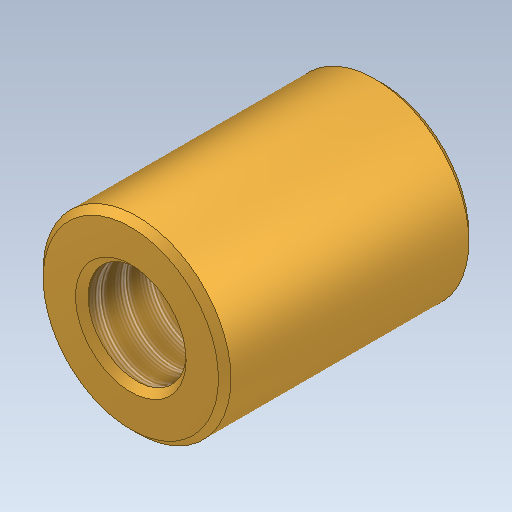
# Autodesk Inventor part: SB-203040
Saved by Autodesk Inventor 2021 (Build 250183000, 183)
## iProperties
Created: 2020-09-13
Part Number: SB-203040
Material: 真鍮、ソフト イエロー
Document SubType Name: Modeling
Designer: Yuta Kage
Mass: 0.173147 g
Surface Area: 0.662651 cm^2
Volume: 0.0204424 cm^3
Density: 8.47 g/cm^3
Appearance: 真鍮 - サテン
Description: 在庫有
Author: Yuta Kage
Autodesk Inventor part; units mm, degrees
ref_plane "YZ Plane" through (0, 0, 0) normal (1, 0, 0) x (0, 1, 0)
ref_plane "XZ Plane" through (0, 0, 0) normal (0, 1, 0) x (-1, 0, 0)
ref_plane "XY Plane" through (0, 0, 0) normal (0, 0, 1) x (1, 0, 0)
sketch "スケッチ1" plane through (0, 0, 0) normal (0, 0, 1) x (1, 0, 0)
  circle A0 centre (0, 0) radius 1.5
  dimension "d0" = 3
  constraints: 1 centre point, 1 coincident
  measures "d0" diameter of A0
extrude "押し出し1" add sketch "スケッチ1" along normal blind 4
sketch "スケッチ2" plane through (0, 0, 4) normal (0, 0, 1) x (1, 0, 0)
  circle A0 centre (0, 0) radius 1.5 construction
hole "穴1" at (0, 0, 4) direction (0, 0, -1) diameter 1.567 end through all thread size "M2x0.4" class "6H" standard "ANSI Metric M Profile"
chamfer "面取り1" distance 0.1 angle 45 3 edges at (0, 0.7835, 4) (-1.5, 0, 4) (-1.5, 0, 0)
